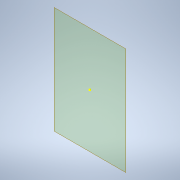
# Autodesk Inventor part: Omniscope_sidewall_spacer_v0
Saved by Autodesk Inventor 2022 (Build 260153000, 153)
## iProperties
Created: 2022-05-27
Part Number: Omniscope_sidewall_spacer_v0
Material: Generisch
Document SubType Name: Modeling
Designer: diederichbenedict
Density: 1 g/cm^3
Appearance: Vorgabe
Author: diederichbenedict
Autodesk Inventor part; units mm, degrees
ref_plane "YZ Plane" through (0, 0, 0) normal (1, 0, 0) x (0, 1, 0)
ref_plane "XZ Plane" through (0, 0, 0) normal (0, 1, 0) x (-1, 0, 0)
ref_plane "XY Plane" through (0, 0, 0) normal (0, 0, 1) x (1, 0, 0)
ref_plane "Arbeitsebene1" through (0, 0, 0) normal (0, 0, -1) x (-1, 0, 0)
sketch "Skizze1" plane through (0, 0, 0) normal (0, 0, -1) x (-1, 0, 0)
  arc A0 (34.75, 57.75) -> (36.75, 55.75) centre (36.75, 57.75) ccw projected
  line L0 (34.75, 57.75) -> (34.75, 60.25) projected
  arc A1 (34.75, 60.25) -> (32.75, 62.25) centre (32.75, 60.25) ccw projected
  line L1 (32.75, 62.25) -> (-32.25, 62.25) projected
  arc A2 (-32.25, 62.25) -> (-34.25, 60.25) centre (-32.25, 60.25) ccw projected
  line L2 (-34.25, 60.25) -> (-34.25, 57.25) projected
  arc A3 (-36.25, 55.25) -> (-34.25, 57.25) centre (-36.25, 57.25) ccw projected
  line L3 (-36.25, 55.25) -> (-39.25, 55.25) projected
  arc A4 (-39.25, 55.25) -> (-41.25, 53.25) centre (-39.25, 53.25) ccw projected
  line L4 (-41.25, 53.25) -> (-41.25, -58.75) projected
  arc A5 (-41.25, -58.75) -> (-37.75, -62.25) centre (-37.75, -58.75) ccw projected
  line L5 (-37.75, -62.25) -> (-33.25, -62.25) projected
  arc A6 (-33.25, -62.25) -> (-31.25, -60.25) centre (-33.25, -60.25) ccw projected
  line L6 (-31.25, -60.25) -> (-31.25, -57.25) projected
  arc A7 (-29.25, -55.25) -> (-31.25, -57.25) centre (-29.25, -57.25) ccw projected
  line L7 (-29.25, -55.25) -> (-26.25, -55.25) projected
  arc A8 (-24.25, -57.25) -> (-26.25, -55.25) centre (-26.25, -57.25) ccw projected
  line L8 (-24.25, -57.25) -> (-24.25, -60.25) projected
  arc A9 (-24.25, -60.25) -> (-22.25, -62.25) centre (-22.25, -60.25) ccw projected
  line L9 (-22.25, -62.25) -> (30.5541, -62.25) projected
  arc A10 (30.5541, -62.25) -> (32.5541, -60.25) centre (30.5541, -60.25) ccw projected
  line L10 (32.5541, -60.25) -> (32.5541, -56.8048) projected
  arc A11 (34.5541, -54.8048) -> (32.5541, -56.8048) centre (34.5541, -56.8048) ccw projected
  line L11 (34.5541, -54.8048) -> (39.25, -54.8048) projected
  arc A12 (39.25, -54.8048) -> (41.25, -52.8048) centre (39.25, -52.8048) ccw projected
  line L12 (41.25, -52.8048) -> (41.25, 53.75) projected
  arc A13 (41.25, 53.75) -> (39.25, 55.75) centre (39.25, 53.75) ccw projected
  line L13 (39.25, 55.75) -> (36.75, 55.75) projected
  line L14 (-42.75, -58.75) -> (-42.75, 58.75) projected
  arc A14 (-37.75, 63.75) -> (-42.75, 58.75) centre (-37.75, 58.75) ccw projected
  line L15 (-37.75, 63.75) -> (37.75, 63.75) projected
  arc A15 (42.75, 58.75) -> (37.75, 63.75) centre (37.75, 58.75) ccw projected
  line L16 (42.75, 58.75) -> (42.75, -58.75) projected
  arc A16 (37.75, -63.75) -> (42.75, -58.75) centre (37.75, -58.75) ccw projected
  line L17 (37.75, -63.75) -> (-37.75, -63.75) projected
  arc A17 (-42.75, -58.75) -> (-37.75, -63.75) centre (-37.75, -58.75) ccw projected
  circle A18 centre (37.75, 58.75) radius 1.4 projected
  circle A19 centre (37.75, -58.75) radius 1.4 projected
  circle A20 centre (-37.75, 58.75) radius 1.4 projected
  circle A21 centre (-28.25, -59.25) radius 1.4 projected
  point P0 (0, 0)
extrude "Extrusion1" add sketch "Skizze1" against normal blind 8.2
